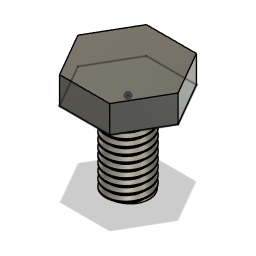
TornilloM8 v1 (Autodesk Fusion 360 design; units mm, degrees)
Autodesk Fusion 360 part; units mm, degrees
sketch "Sketch1" plane through (0, 0, 0) normal (0, 1, 0) x (1, 0, 0)
  circle A0 centre (0, 0) radius 3.8
  dimension "d1" = 7.6
  constraint coincident A0.centre origin
  measures "d1" diameter of A0
extrude "Extrude1" add sketch "Sketch1" along normal blind 15
thread "Thread1" "ISO Metric profile 8.0 M8x1.25 6g" major diameter 7.866 minor diameter 6.4455 pitch 1.25 angle 60 modelled right hand crest width 0.1833 on face at (3.7811, 10, 0.3784) crest through (3.933, -0.3125, 0)
sketch "Sketch2" plane through (0, 15, 0) normal (0, 1, 0) x (-1, 0, 0)
  line L0 (-9.2376, 0) -> (-4.6188, -8)
  line L1 (-4.6188, -8) -> (4.6188, -8)
  line L2 (4.6188, -8) -> (9.2376, 0)
  line L3 (9.2376, 0) -> (4.6188, 8)
  line L4 (4.6188, 8) -> (-4.6188, 8)
  line L5 (-4.6188, 8) -> (-9.2376, 0)
  dimension "d8" = 8
  constraint horizontal L1
  measures "d8" distance of origin L5
extrude "Extrude3" add sketch "Sketch2" along normal blind 5
